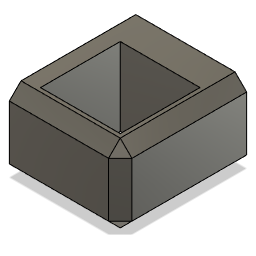
Hanger__Rod (Autodesk Fusion 360 design; units mm, degrees)
Autodesk Fusion 360 part; units mm, degrees
sketch "Sketch1" plane through (0, 0, 0) normal (0, 1, 0) x (1, 0, 0)
  line L0 (0, 0) -> (20.5, 0)
  line L1 (20.5, 0) -> (20.5, -20.5)
  line L2 (20.5, -20.5) -> (0, -20.5)
  line L3 (0, -20.5) -> (0, 0)
  line L4 (0, 0) -> (-4, 0)
  line L5 (-4, 0) -> (-4, 4)
  line L6 (-4, 4) -> (0, 4)
  line L7 (0, 4) -> (0, 0)
  line L8 (-4, 4) -> (24.5, 4)
  line L9 (24.5, 4) -> (24.5, -24.5)
  line L10 (24.5, -24.5) -> (-4, -24.5)
  line L11 (-4, -24.5) -> (-4, 4)
  dimension "d1" = 20.5
  dimension "d2" = 20.5
  dimension "d3" = 4
  dimension "d4" = 4
  dimension "d5" = 28.5
  dimension "d6" = 28.5
  constraint horizontal L0
  constraint vertical L1
  constraint horizontal L2
  constraint vertical L3
  constraint coincident L0.start L3.end
  constraint horizontal L4
  constraint vertical L5
  constraint horizontal L6
  constraint vertical L7
  constraint horizontal L8
  constraint vertical L9
  constraint horizontal L10
  constraint vertical L11
  measures "d1" distance of L0.start L0.end
  measures "d2" distance of L0.start L2.end
  measures "d3" distance of L0.start L4.end
  measures "d4" distance of L0.start L6.end
  measures "d5" distance of L5.end L8.end
  measures "d6" distance of L5.end L10.end
extrude "Extrude1" add sketch "Sketch1" along normal blind 20
chamfer "Chamfer1" distance 3 angle 45 5 edges at (24.5, 20, 10.25) (10.25, 20, 24.5) (24.5, 10, 24.5) (24.5, 0, 10.25) (10.25, 0, 24.5)
sketch "Sketch2" plane through (0, 0, -4) normal (0, 0, -1) x (-1, 0, 0)
  line L0 (-24.5, 3) -> (-21.5, 0)
  line L1 (-21.5, 0) -> (4, 0)
  line L2 (4, 0) -> (4, 20)
  line L3 (4, 20) -> (-21.5, 20)
  line L4 (-21.5, 20) -> (-24.5, 17)
  line L5 (-24.5, 17) -> (-24.5, 3)
  line L6 (-24.5, 10) -> (-10.25, 10)
  line L7 (-7.6519, 5.5) -> (-5.0538, 10)
  line L8 (-5.0538, 10) -> (-7.6519, 14.5)
  line L9 (-7.6519, 14.5) -> (-12.8481, 14.5)
  line L10 (-12.8481, 14.5) -> (-15.4462, 10)
  line L11 (-15.4462, 10) -> (-12.8481, 5.5)
  line L12 (-12.8481, 5.5) -> (-7.6519, 5.5)
  point P0 (-10.25, 10)
  dimension "d10" = 14.25
  dimension "d11" = 4.5
  constraint midpoint L5 L6.start
  constraint perpendicular L2 L6
  constraint coincident P0 L6.end
  measures "d10" distance of L6.start P0
  measures "d11" distance of P0 L12
extrude "Extrude2" add sketch "Sketch2" along normal blind 4
